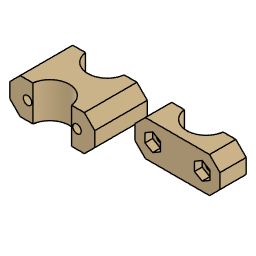
Cunha em H e C v2 (Autodesk Fusion 360 design; units mm, degrees)
Autodesk Fusion 360 part; units mm, degrees
sketch "Sketch1" plane through (0, 0, 0) normal (0, 1, 0) x (1, 0, 0)
  circle A0 centre (0, 0) radius 2.75
  circle A1 centre (32, 0) radius 2.75
  line L0 (0, 0) -> (32, 0) construction
  line L1 (0, -11.5) -> (32, -11.5)
  arc A2 (32, -11.5) -> (32, 11.5) centre (32, 0) ccw
  line L2 (32, 11.5) -> (0, 11.5)
  arc A3 (0, 11.5) -> (0, -11.5) centre (0, 0) ccw
  line L3 (-5, -2.8868) -> (0, -5.7735)
  line L4 (0, -5.7735) -> (5, -2.8868)
  line L5 (5, -2.8868) -> (5, 2.8868)
  line L6 (5, 2.8868) -> (0, 5.7735)
  line L7 (0, 5.7735) -> (-5, 2.8868)
  line L8 (-5, 2.8868) -> (-5, -2.8868)
  line L9 (37, 2.8868) -> (32, 5.7735)
  line L10 (32, 5.7735) -> (27, 2.8868)
  line L11 (27, 2.8868) -> (27, -2.8868)
  line L12 (27, -2.8868) -> (32, -5.7735)
  line L13 (32, -5.7735) -> (37, -2.8868)
  line L14 (37, -2.8868) -> (37, 2.8868)
  line L15 (0, -11.5) -> (-8.8382, -7.3577)
  line L16 (-11.5, 0) -> (-11.5, 4.7635)
  line L17 (-11.5, 4.7635) -> (-4.7635, 11.5)
  line L18 (-4.7635, 11.5) -> (0, 11.5)
  line L19 (-11.5, 0) -> (-11.5, -4.7635)
  line L20 (-11.5, -4.7635) -> (-4.7635, -11.5)
  line L21 (-4.7635, -11.5) -> (0, -11.5)
  line L22 (16, 0) -> (16, -11.5) construction
  line L23 (43.5, 0) -> (43.5, -4.7635)
  line L24 (43.5, -4.7635) -> (36.7635, -11.5)
  line L25 (36.7635, -11.5) -> (32, -11.5)
  line L26 (43.5, 4.7635) -> (36.7635, 11.5)
  line L27 (36.7635, 11.5) -> (32, 11.5)
  line L28 (43.5, 0) -> (43.5, 4.7635)
  point P0 (32, 0)
  dimension "d1" = 5.5
  dimension "d2" = 32
  dimension "d3" = 23
  dimension "d4" = 10
  dimension "d11" = 135
  constraint coincident A0.centre L0.start
  constraint coincident P0 A1.centre
  constraint horizontal L0
  constraint equal A0 A1
  constraint horizontal L1
  constraint tangent L1 A2
  constraint tangent A2 L2
  constraint parallel L1 L2
  constraint tangent L2 A3
  constraint tangent L1 A3
  constraint vertical L5
  constraint vertical L11
  constraint equal L4 L12
  constraint coincident A3 L15.end
  constraint midpoint A3 L16.start
  constraint tangent A3 L16
  constraint vertical L16
  constraint horizontal L18
  constraint tangent A3 L17
  constraint symmetric L0 L2.end L1.start
  constraint symmetric L0 L16.start L19.start
  constraint symmetric L0 L16.end L19.end
  constraint symmetric L0 L17.end L20.end
  constraint midpoint L0 L22.start
  constraint midpoint L1 L22.end
  constraint symmetric L2.end L22 A2.end
  constraint symmetric L16.start L22 L23.start
  constraint symmetric L16.end L22 L26.start
  constraint symmetric L17.end L22 L26.end
  constraint symmetric L19.end L22 L23.end
  constraint symmetric L20.end L22 L24.end
  constraint symmetric L1.start L22 L1.end
  measures "d1" diameter of A1
  measures "d2" distance of A0.centre P0
  measures "d3" distance of L1 L2
  measures "d4" distance of L3 L6
  measures "d11" angle of L17 L18
extrude "Extrude1" add sketch "Sketch1" along normal blind 17 contours L1 A2 L2 A3 L15 | A3 L20 L21 | A3 L15 | A2 L24 L25 | A3 L19 L20 | A2 L23 L24 | A3 L16 L17 | A2 L26 L28 | A3 L17 L18 | A2 L26 L27 makes body 1
extrude "Extrude2" add sketch "Sketch1" along normal up to surface (12 mm away) from surface at 5 contours L3 L4 L5 L6 L7 L8 | L9 L10 L11 L12 L13 L14 bodies 1
sketch "Sketch2" plane through (0, 0, 11.5) normal (0, 0, 1) x (-1, 0, 0)
  line L0 (4.7635, 0) -> (-36.7635, 0)
  line L1 (-36.7635, 0) -> (-36.7635, -17)
  line L2 (-36.7635, -17) -> (4.7635, -17)
  line L3 (4.7635, -17) -> (4.7635, 0)
  arc A0 (-3.5, -17) -> (-28.5, -17) centre (-16, -18.6023) ccw
  line L4 (-16, -17) -> (-16, -6) construction
  line L5 (-3.5, -17) -> (-28.5, -17)
  dimension "d12" = 25
  dimension "d14" = 11
  constraint midpoint L2 L4.start
  constraint midpoint A0 L4.end
  constraint vertical L4
  constraint horizontal L5
  constraint coincident L4.start L5
  measures "d12" distance of A0.start A0.end
  measures "d14" distance of L4.start L4.end
extrude "Extrude3" cut sketch "Sketch2" against normal through all contours L2 A0 L5 bodies 1
copy_body "CopyPasteBodies1" bodies 1 makes body 2
move_body "Move1" bodies 2 to x (1, 0, 0) y (0, 1, 0) z (0, 0, 1) at (64, 0, 0)
extrude "Extrude4" add 2 faces at (29.875, 5, 3.6806) (-2.125, 5, 3.6806) along direction (0, -1, 0) up to surface end surface through (0, 0, 0) normal (0, -1, 0) offset 0 on bodies 1 bodies 1
mirror "Mirror1" about plane through (0, 0, 0) normal (0, -1, 0) of bodies 1 merged
